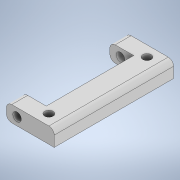
# Autodesk Inventor part: krepleniye
Saved by Autodesk Inventor 2020 (Build 240168000, 168)
## iProperties
Created: 2022-07-21
Part Number: krepleniye
Material: Типовые
Document SubType Name: Modeling
Designer: akapu
Density: 1 g/cm^3
Appearance: По умолчанию
Author: akapu
Autodesk Inventor part; units mm, degrees
ref_plane "YZ Plane" through (0, 0, 0) normal (1, 0, 0) x (0, 1, 0)
ref_plane "XZ Plane" through (0, 0, 0) normal (0, 1, 0) x (-1, 0, 0)
ref_plane "XY Plane" through (0, 0, 0) normal (0, 0, 1) x (1, 0, 0)
sketch "Эскиз1" plane through (0, 0, 0) normal (0, 1, 0) x (-1, 0, 0)
  line L0 (0, 0) -> (-8, 0)
  line L1 (-8, 0) -> (-8, -37)
  line L2 (-8, -37) -> (0, -37)
  line L3 (0, -37) -> (0, 0)
  circle A0 centre (-8, 0) radius 1.6
  line L4 (-8, -37) -> (-2, -37)
  line L5 (-2, -37) -> (-2, -41)
  line L6 (-2, -41) -> (-14, -41)
  line L7 (-14, -41) -> (-14, 4)
  line L8 (-14, 4) -> (0, 4)
  line L9 (0, 4) -> (0, 0)
  line L10 (-2, -41) -> (0, -41)
  line L11 (0, -41) -> (0, -37)
  line L12 (0, 4) -> (4, 4)
  line L13 (4, 4) -> (4, -41)
  line L14 (4, -41) -> (0, -41)
  line L15 (0, -41) -> (0, 4)
  line L16 (4, 4) -> (4, -2)
  line L17 (4, -2) -> (-2, -2)
  line L18 (-2, -2) -> (-2, -37)
  line L19 (4, -41) -> (4, -35)
  line L20 (4, -35) -> (-2, -35)
  circle A1 centre (-8, -37) radius 1.6
  dimension "d0" = 8
  dimension "d1" = 37
  dimension "d2" = 3.2
  dimension "d4" = 6
  dimension "d5" = 4
  dimension "d6" = 12
  dimension "d7" = 45
  dimension "d10" = 4
  dimension "d13" = 6
  dimension "d14" = 6
  dimension "d15" = 6
  dimension "d28" = 3.2
  constraints: 42 end point, 10 perpendicular, 5 point on line, 4 parallel, 3 coincident, 2 centre point, 2 horizontal, 1 vertical
  measures "d0" distance of L2.end L1.end
  measures "d1" distance of L1.end L0.end
  measures "d2" diameter of A0
  measures "d4" distance of L4.start L4.end
  measures "d5" distance of L4.end L5.end
  measures "d6" distance of L5.end L6.end
  measures "d7" distance of L6.end L7.end
  measures "d10" distance of L13.end L14.end
  measures "d13" distance of L12.end L16.end
  measures "d14" distance of L16.end L17.end
  measures "d15" distance of L13.end L19.end
  measures "d28" diameter of A1
extrude "Выдавливание1" add sketch "Эскиз1" along normal blind 6 contours L3 L17 L18 L2 A1 L1 A0 L0 | L9 L12 L13 L17 L3 | L0 A0 L1 A1 L2 L5 L6 L7 L8 L9 | L20 L13 L14 L11 L3 | L3 L2 L18 L20 | L11 L10 L5 L2
sketch "Эскиз3" plane through (-4, 0, 4) normal (0, 0, 1) x (1, 0, 0)
  line L0 (0, 0) -> (18, 0) projected
  line L1 (0, 0) -> (4, 0)
  line L2 (4, 0) -> (4, 3)
  line L3 (4, 3) -> (0, 3)
  line L4 (0, 3) -> (0, 0)
  circle A0 centre (4, 3) radius 1.6
  dimension "d16" = 4
  dimension "d17" = 3
  dimension "d18" = 3.2
  constraints: 8 end point, 2 parallel, 1 centre point, 1 coincident, 1 horizontal, 1 perpendicular
  measures "d16" distance of L3.end L2.end
  measures "d17" distance of L2.end L1.end
  measures "d18" diameter of A0
extrude "Выдавливание2" cut sketch "Эскиз3" against normal blind 45 contours A0 L3 L2 | L2 L3 A0
fillet "Сопряжение2" radius 2 5 edges at (-4, 6, 1) (-4, 6, -38) (-4, 0, -38) (-4, 0, 1) (14, 6, -18.5)
sketch "Эскиз5" plane through (2, 0, -2) normal (0, 0, -1) x (-1, 0, 0)
  line L0 (0, 0) -> (0, 6) projected
  line L1 (0, 0) -> (6.2917, 0) construction
  line L2 (0, 0) -> (-3.4641, 6)
  line L3 (-10, 6) -> (4, 6) projected
  line L4 (0, 0) -> (6.9282, 0) construction
  line L5 (0, 6) -> (-3, 6)
  line L6 (-3, 6) -> (0, 0)
  line L7 (0, 0) -> (0, 6)
  point P0 (2, 0)
  dimension "d24" = 120
  dimension "d25" = 3
  constraints: 12 end point, 2 horizontal, 1 collinear, 1 equal length, 1 midpoint, 1 point on line
  measures "d24" angle of L4 L2
  measures "d25" distance of L0.end L5.end
extrude "Выдавливание3" cut sketch "Эскиз5" along normal blind 33 contours L6 L3 L0
